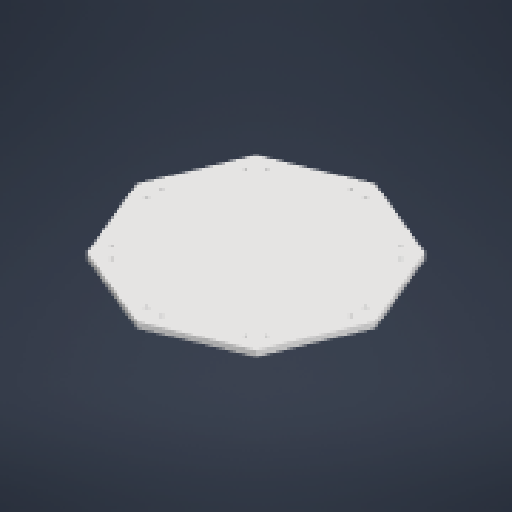
# Autodesk Inventor part: Bund
Saved by Autodesk Inventor 2026.1 (Build 301233020, 233B)
## iProperties
Created: 2026-04-22
Part Number: Bund
Material: Generic
Document SubType Name: Modeling
Designer: Mikke
Density: 1 g/cm^3
Appearance: Default
Author: Mikke
Autodesk Inventor part; units mm, degrees
ref_plane "YZ Plane" through (0, 0, 0) normal (1, 0, 0) x (0, 1, 0)
ref_plane "XZ Plane" through (0, 0, 0) normal (0, 1, 0) x (-1, 0, 0)
ref_plane "XY Plane" through (0, 0, 0) normal (0, 0, 1) x (1, 0, 0)
sketch "Sketch1" plane through (0, 0, 0) normal (0, 1, 0) x (-1, 0, 0)
  line L0 (0, 0) -> (0, -104.6)
  line L1 (0, -104.6) -> (-73.9634, -73.9634)
  line L2 (-73.9634, -73.9634) -> (-104.6, 0)
  line L3 (-104.6, 0) -> (-73.9634, 73.9634)
  line L4 (-73.9634, 73.9634) -> (0, 104.6)
  line L5 (0, 104.6) -> (73.9634, 73.9634)
  line L6 (73.9634, 73.9634) -> (104.6, 0)
  line L7 (104.6, 0) -> (73.9634, -73.9634)
  line L8 (73.9634, -73.9634) -> (0, -104.6)
  line L9 (89.2707, -89.2707) -> (126.2478, 0)
  line L10 (126.2478, 0) -> (89.2707, 89.2707)
  line L11 (89.2707, 89.2707) -> (0, 126.2478)
  line L12 (0, 126.2478) -> (-89.2707, 89.2707)
  line L13 (-89.2707, 89.2707) -> (-126.2478, 0)
  line L14 (-126.2478, 0) -> (-89.2707, -89.2707)
  line L15 (-89.2707, -89.2707) -> (0, -126.2478)
  line L16 (0, -126.2478) -> (89.2707, -89.2707)
  line L17 (0, -104.6) -> (7.6537, -123.0776)
  line L18 (0, -104.6) -> (20, -104.6) construction
  line L19 (73.9634, -73.9634) -> (81.617, -92.441)
  line L20 (73.9634, -73.9634) -> (76.2595, -79.5066)
  line L21 (76.2595, -79.5066) -> (70.7162, -81.8027)
  circle A0 centre (70.7162, -81.8027) radius 1.6
  line L22 (0, -104.6) -> (2.2961, -110.1433)
  line L23 (2.2961, -110.1433) -> (7.8394, -107.8472)
  circle A1 centre (7.8394, -107.8472) radius 1.6
  circle A2 centre (107.8472, -7.8394) radius 1.6
  circle A3 centre (81.8027, -70.7162) radius 1.6
  circle A4 centre (81.8027, 70.7162) radius 1.6
  circle A5 centre (107.8472, 7.8394) radius 1.6
  circle A6 centre (7.8394, 107.8472) radius 1.6
  circle A7 centre (70.7162, 81.8027) radius 1.6
  circle A8 centre (-70.7162, 81.8027) radius 1.6
  circle A9 centre (-7.8394, 107.8472) radius 1.6
  circle A10 centre (-107.8472, 7.8394) radius 1.6
  circle A11 centre (-81.8027, 70.7162) radius 1.6
  circle A12 centre (-81.8027, -70.7162) radius 1.6
  circle A13 centre (-107.8472, -7.8394) radius 1.6
  circle A14 centre (-7.8394, -107.8472) radius 1.6
  circle A15 centre (-70.7162, -81.8027) radius 1.6
  dimension "d0" = 104.6
  dimension "d1" = 20
  dimension "d2" = 67.5
  dimension "d3" = 6
  dimension "d4" = 6
  dimension "d5" = 3.2
  dimension "d6" = 6
  dimension "d7" = 3.2
  dimension "d10" = 360
  constraints: 48 end point, 16 centre point, 4 point on line, 3 coincident, 3 perpendicular, 1 equal length, 1 horizontal, 1 vertical, 57 other
  measures "d0" distance of L0.start L0.end
  measures "d1" distance between parallel lines of L7 L9
  measures "d2" angle of L17 L18
  measures "d3" distance of L7.end L20.end
  measures "d4" distance of L20.end L21.end
  measures "d5" diameter of A0
  measures "d6" distance of L22.end L23.end
  measures "d7" diameter of A1
extrude "Extrusion1" add sketch "Sketch1" along normal blind 6
body "Solid1"
